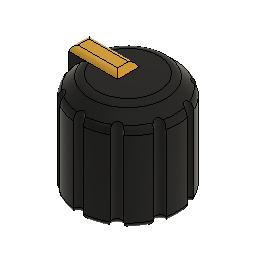
cace_assembly (Autodesk Fusion 360 archive; units mm, degrees)
design "deej knob"
Autodesk Fusion 360 part; units mm, degrees
sketch "Sketch1" plane through (0, 0, 0) normal (0, 0, 1) x (1, 0, 0)
  circle A0 centre (0, 0) radius 3.1
  circle A1 centre (0, 0) radius 5
  circle A2 centre (0, 0) radius 3
  circle A3 centre (0, 5) radius 0.5
  circle A4 centre (-2.9389, 4.0451) radius 0.5
  circle A5 centre (-4.7553, 1.5451) radius 0.5
  circle A6 centre (-4.7553, -1.5451) radius 0.5
  circle A7 centre (-2.9389, -4.0451) radius 0.5
  circle A8 centre (0, -5) radius 0.5
  circle A9 centre (2.9389, -4.0451) radius 0.5
  circle A10 centre (4.7553, -1.5451) radius 0.5
  circle A11 centre (4.7553, 1.5451) radius 0.5
  circle A12 centre (2.9389, 4.0451) radius 0.5
  line L0 (0, 0) -> (0, 1.0451)
  line L1 (0, 1.0451) -> (-4.8896, 1.0451)
  line L2 (0, 0) -> (0, -1.0451)
  line L3 (0, -1.0451) -> (-4.8896, -1.0451)
  dimension "d1" = 6.2
  dimension "d2" = 10
  dimension "d3" = 6
  dimension "d4" = 1
  dimension "d6" = 360
  constraint coincident A0.centre A1.centre
  constraint concentric A0 A1
  constraint concentric A0 A2
  constraint coincident A1 A3.centre
  constraint vertical L0
  constraint horizontal L1
  constraint vertical L2
  constraint horizontal L3
  constraint coincident A1 L1.end
  constraint coincident A1 L3.end
  constraint tangent A6 L3
  constraint tangent A5 L1
  measures "d1" diameter of A0
  measures "d2" diameter of A1
  measures "d3" diameter of A2
  measures "d4" diameter of A3
extrude "Extrude1" add sketch "Sketch1" along normal blind 9 contours A0 A1 A3 A4 A5 A6 A7 A8 A9 A10 A11 A12 L1 L3 | A0 A1 L1 L3 | A1 A5 L1 | A1 A6 L3
extrude "Extrude2" add sketch "Sketch1" along normal blind 9 and the other way blind -4 contours A0 A2 L1 L3 | A0 A2 L1 L3
extrude "Extrude3" add sketch "Sketch1" along normal blind 1 from surface at 9 contours A0 A2 L1 L3 | A0 A1 A3 A4 A5 A6 A7 A8 A9 A10 A11 A12 L1 L3 | A0 A2 L1 L3 | A0 A1 L1 L3 | A2 L0 L1 L2 L3 | A2 L0 L1 L2 L3 | A1 A5 L1 | A1 A6 L3
sketch "Sketch2" plane through (0, 0, 0) normal (1, 0, 0) x (0, 1, 0)
  line L0 (-5.5, 8) -> (-3, 10.5)
  line L1 (-3, 10.5) -> (-5.5, 10.5)
  line L2 (-5.5, 10.5) -> (-5.5, 8)
  dimension "d26" = 8
  dimension "d27" = 3
  constraint horizontal L1
  constraint perpendicular L1 L2
  measures "d26" vertical distance of origin L0.start
  measures "d27" horizontal distance of origin L0.end
revolve "Revolve1" cut sketch "Sketch2" angle 360 about axis through (0, 0, 1.75) along (0, 0, 1)
fillet "Fillet4" radius 1 1 edges at (-1.2657, 3.2631, 10)
fillet "Fillet5" radius 1 10 edges at (4.0451, 2.9389, 8.5) (1.5451, 4.7553, 8.5) (-1.5451, 4.7553, 8.5) (-4.0451, 2.9389, 8.5) (-5, 0, 8.5) (-4.0451, -2.9389, 8.5) (-1.5451, -4.7553, 8.5) (1.5451, -4.7553, 8.5) (4.0451, -2.9389, 8.5) (5, 0, 8.5)
extrude "Extrude4" add sketch "Sketch1" along normal blind 10.5 and the other way blind -7.5 contours A0 A2 L1 L3 | A0 A1 L1 L3 | A2 L0 L1 L2 L3 picked at (-2.8875, 0.9086) picked at (-0.9374, 0.6967)
fillet "Fillet6" radius 0.5 4 edges at (-5, 0, 10.5) (-2.4448, -1.0451, 10.5) (0, 0, 10.5) (-2.4448, 1.0451, 10.5)
fillet "Fillet7" radius 0.5 1 faces at (4.2069, -0.4845, 0)

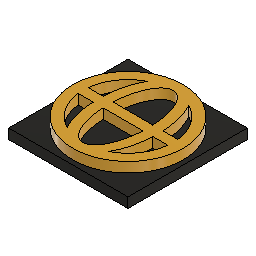
design "www"
Autodesk Fusion 360 part; units mm, degrees
sketch "Sketch1" plane through (0, 0, 0) normal (0, 0, 1) x (1, 0, 0)
  line L0 (5.95, -5.95) -> (-5.95, -5.95)
  line L1 (-5.95, -5.95) -> (-5.95, 5.95)
  line L2 (-5.95, 5.95) -> (5.95, 5.95)
  line L3 (5.95, 5.95) -> (5.95, -5.95)
  line L4 (5.95, -5.95) -> (-5.95, 5.95) construction
  line L5 (-5.95, -5.95) -> (5.95, 5.95) construction
  circle A0 centre (0, 0) radius 5.5
  arc A1 (-2.058, 4.0018) -> (-4.4755, 0.4687) centre (0, 0) ccw
  arc A2 (-4.4755, -0.4687) -> (-2.058, -4.0018) centre (0, 0) ccw
  ellipse E0 centre (0, 0) end of major axis (3, 0) minor radius 5.5 (-2.058, 4.0018) -> (-2.9876, 0.5) ccw
  ellipse E1 centre (0, 0) end of major axis (3, 0) minor radius 5.5 (-2.9876, -0.5) -> (-2.058, -4.0018) ccw
  arc A3 (2.058, -4.0018) -> (4.4721, -0.5) centre (0, 0) ccw
  arc A4 (4.4721, 0.5) -> (2.058, 4.0018) centre (0, 0) ccw
  line L6 (2.9876, 0.5) -> (4.4721, 0.5)
  ellipse E2 centre (0, 0) end of major axis (3, 0) minor radius 5.5 (2.058, -4.0018) -> (2.9876, -0.5) ccw
  ellipse E3 centre (0, 0) end of major axis (3, 0) minor radius 5.5 (2.9876, 0.5) -> (2.058, 4.0018) ccw
  ellipse E4 centre (0, 0) end of major axis (2, 0) minor radius 4.5 (-1.9876, -0.5) -> (1.9876, -0.5) ccw
  ellipse E5 centre (0, 0) end of major axis (2, 0) minor radius 4.5 (1.9876, 0.5) -> (-1.9876, 0.5) ccw
  line L7 (4.4721, -0.5) -> (2.9876, -0.5)
  line L8 (1.9876, -0.5) -> (-1.9876, -0.5)
  line L9 (-2.9876, -0.5) -> (-4.4721, -0.5)
  line L10 (-4.4721, 0.5) -> (-2.9876, 0.5)
  line L11 (-1.9876, 0.5) -> (1.9876, 0.5)
  dimension "d1" = 11.9
  dimension "d2" = 11.9
  constraint horizontal L0
  constraint perpendicular L0 L1
  constraint parallel L0 L2
  constraint parallel L1 L3
  constraint concentric A0 A1
  constraint concentric A0 E0
  constraint concentric A1 A3
  constraint coincident A3.start E0
  constraint concentric E0 E2
  constraint horizontal L7
  constraint parallel L7 L10
  constraint coincident A0.centre A1.centre
  constraint coincident L10.start A1
  constraint coincident L9.end A1
  constraint coincident A2.start A1
  constraint concentric A1 A2
  constraint concentric E0 E1
  constraint coincident L11.start L10
  constraint coincident L8.end L7
  constraint coincident L9.start L7
  constraint coincident A4.start A3
  constraint concentric A3 A4
  constraint coincident L11.end E4
  constraint coincident L6.start E2
  constraint collinear L6 L10
  constraint concentric E2 E3
  constraint coincident L8.start L7
  constraint concentric E4 E5
  constraint collinear L7 L8
  constraint collinear L8 L9
  constraint collinear L10 L11
  measures "d1" distance of L1.end L2.end
  measures "d2" distance of L0.end L1.end
extrude "Extrude1" add sketch "Sketch1" against normal blind 1 contours L0 L1 L2 L3 | A0 | A1 E0 L10 | A2 E1 L9 | A3 E2 L7 | A4 L6 E3 | E4 L8 | E5 L11
extrude "Extrude3" add sketch "Sketch1" along normal blind 1 contours A0

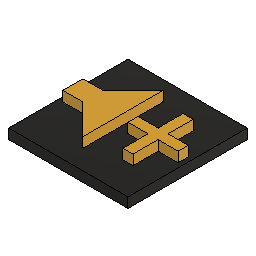
design "volume"
Autodesk Fusion 360 part; units mm, degrees
sketch "Sketch1" plane through (0, 0, 0) normal (0, 0, 1) x (1, 0, 0)
  line L0 (5.95, -5.95) -> (-5.95, -5.95)
  line L1 (-5.95, -5.95) -> (-5.95, 5.95)
  line L2 (-5.95, 5.95) -> (5.95, 5.95)
  line L3 (5.95, 5.95) -> (5.95, -5.95)
  line L4 (5.95, -5.95) -> (-5.95, 5.95) construction
  line L5 (-5.95, -5.95) -> (5.95, 5.95) construction
  line L6 (-0.5, 3.5) -> (-0.5, 0)
  line L7 (0.5, 0) -> (0.5, 0.5)
  line L8 (2.5, 3) -> (3.5, 3)
  line L9 (5.5, 0.5) -> (5.5, -0.5)
  line L10 (3.5, -3) -> (2.5, -3)
  line L11 (0.5, 0) -> (0.5, -0.5)
  line L12 (0.5, 0.5) -> (2.5, 0.5)
  line L13 (2.5, 0.5) -> (2.5, 3)
  line L14 (3.5, 3) -> (3.5, 0.5)
  line L15 (3.5, 0.5) -> (5.5, 0.5)
  line L16 (5.5, -0.5) -> (3.5, -0.5)
  line L17 (3.5, -0.5) -> (3.5, -3)
  line L18 (2.5, -3) -> (2.5, -0.5)
  line L19 (2.5, -0.5) -> (0.5, -0.5)
  line L20 (-0.5, 0) -> (-0.5, -3.5)
  line L21 (-3.5, -1) -> (-5.5, -1)
  line L22 (-5.5, -1) -> (-5.5, 1)
  line L23 (-5.5, 1) -> (-3.5, 1)
  line L24 (-0.5, 3.5) -> (-0.5, 4)
  line L25 (-0.5, 4) -> (-3.5, 1)
  line L26 (-0.5, -3.5) -> (-0.5, -4)
  line L27 (-0.5, -4) -> (-3.5, -1)
  dimension "d1" = 11.9
  dimension "d2" = 11.9
  constraint horizontal L0
  constraint perpendicular L0 L1
  constraint parallel L0 L2
  constraint parallel L1 L3
  constraint coincident L4 origin
  constraint coincident L5 origin
  constraint parallel L1 L7
  constraint perpendicular L7 L12
  constraint perpendicular L8 L13
  constraint perpendicular L9 L15
  constraint perpendicular L9 L16
  constraint perpendicular L10 L17
  constraint perpendicular L10 L18
  constraint perpendicular L11 L19
  constraint parallel L6 L20
  constraint perpendicular L20 L21
  constraint perpendicular L21 L22
  constraint perpendicular L22 L23
  constraint parallel L6 L24
  constraint perpendicular L4 L25
  constraint parallel L24 L26
  constraint perpendicular L5 L27
  measures "d1" distance of L1.end L2.end
  measures "d2" distance of L0.end L1.end
extrude "Extrude1" add sketch "Sketch1" against normal blind 1 contours L0 L1 L2 L3 | L6 L20 L21 L22 L23 L24 L25 L26 L27 | L7 L8 L9 L10 L11 L12 L13 L14 L15 L16 L17 L18 L19
extrude "Extrude2" add sketch "Sketch1" along normal blind 1 contours L6 L20 L21 L22 L23 L24 L25 L26 L27 | L7 L8 L9 L10 L11 L12 L13 L14 L15 L16 L17 L18 L19

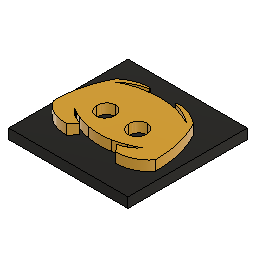
design "discord"
Autodesk Fusion 360 part; units mm, degrees
sketch "Sketch1" plane through (0, 0, 0) normal (0, 0, 1) x (1, 0, 0)
  line L0 (5.95, -5.95) -> (-5.95, -5.95)
  line L1 (-5.95, -5.95) -> (-5.95, 5.95)
  line L2 (-5.95, 5.95) -> (5.95, 5.95)
  line L3 (5.95, 5.95) -> (5.95, -5.95)
  line L4 (5.95, -5.95) -> (-5.95, 5.95) construction
  line L5 (-5.95, -5.95) -> (5.95, 5.95) construction
  spline S0 degree 3 poles (1.569, 0.3676) (1.0713, 0.3676) (0.6784, -0.0602) (0.6784, -0.5928) knots 0 0 0 0 1 1 1 1
  spline S1 degree 3 poles (0.6784, -0.5928) (0.6784, -1.1254) (1.08, -1.5532) (1.569, -1.5532) knots 0 0 0 0 1 1 1 1
  spline S2 degree 3 poles (1.569, -1.5532) (2.0667, -1.5532) (2.4596, -1.1254) (2.4596, -0.5928) knots 0 0 0 0 1 1 1 1
  spline S3 degree 3 poles (2.4596, -0.5928) (2.4596, -0.0602) (2.0579, 0.3676) (1.569, 0.3676) knots 0 0 0 0 1 1 1 1
  spline S4 degree 3 poles (-1.6179, 0.3676) (-2.1156, 0.3676) (-2.5085, -0.0602) (-2.5085, -0.5928) knots 0 0 0 0 1 1 1 1
  spline S5 degree 3 poles (-2.5085, -0.5928) (-2.5085, -1.1254) (-2.1069, -1.5532) (-1.6179, -1.5532) knots 0 0 0 0 1 1 1 1
  spline S6 degree 3 poles (-1.6179, -1.5532) (-1.1202, -1.5532) (-0.7273, -1.1254) (-0.7273, -0.5928) knots 0 0 0 0 1 1 1 1
  spline S7 degree 3 poles (-0.7273, -0.5928) (-0.7186, -0.0602) (-1.1202, 0.3676) (-1.6179, 0.3676) knots 0 0 0 0 1 1 1 1
  spline S8 degree 2 poles (2.4421, -3.6749) (2.1278, -3.2995) (1.8659, -2.9764) knots 0 0 0 1 1 1
  spline S9 degree 2 poles (1.8659, -2.9764) (3.0096, -2.6534) (3.4462, -1.9461) knots 0 0 0 1 1 1
  spline S10 degree 3 poles (3.4462, -1.9461) (3.0882, -2.1819) (2.7477, -2.3478) (2.4421, -2.4613) knots 0 0 0 0 1 1 1 1
  spline S11 degree 3 poles (2.4421, -2.4613) (2.0056, -2.6446) (1.5865, -2.7581) (1.1761, -2.8367) knots 0 0 0 0 1 1 1 1
  spline S12 degree 3 poles (1.1761, -2.8367) (0.3379, -2.9939) (-0.4305, -2.9502) (-1.0853, -2.828) knots 0 0 0 0 1 1 1 1
  spline S13 degree 3 poles (-1.0853, -2.828) (-1.583, -2.7319) (-2.0108, -2.601) (-2.3688, -2.4525) knots 0 0 0 0 1 1 1 1
  spline S14 degree 3 poles (-2.3688, -2.4525) (-2.5696, -2.374) (-2.7879, -2.2779) (-3.0062, -2.1557) knots 0 0 0 0 1 1 1 1
  spline S15 degree 3 poles (-3.0062, -2.1557) (-3.0324, -2.1382) (-3.0586, -2.1295) (-3.0848, -2.112) knots 0 0 0 0 1 1 1 1
  spline S16 degree 3 poles (-3.0848, -2.112) (-3.1022, -2.1033) (-3.111, -2.0946) (-3.1197, -2.0946) knots 0 0 0 0 1 1 1 1
  spline S17 degree 2 poles (-3.1197, -2.0946) (-3.2769, -2.0073) (-3.3642, -1.9461) knots 0 0 0 1 1 1
  spline S18 degree 2 poles (-3.3642, -1.9461) (-2.9451, -2.6359) (-1.8362, -2.9677) knots 0 0 0 1 1 1
  spline S19 degree 2 poles (-1.8362, -2.9677) (-2.0981, -3.2995) (-2.4212, -3.6837) knots 0 0 0 1 1 1
  spline S20 degree 2 poles (-2.4212, -3.6837) (-4.3508, -3.6225) (-5.0842, -2.3652) knots 0 0 0 1 1 1
  spline S21 degree 2 poles (-5.0842, -2.3652) (-5.0842, 0.42) (-3.8269, 2.6814) knots 0 0 0 1 1 1
  spline S22 degree 2 poles (-3.8269, 2.6814) (-2.5696, 3.6157) (-1.3822, 3.5895) knots 0 0 0 1 1 1
  line L6 (-1.3822, 3.5895) -> (-1.2949, 3.4847)
  spline S23 degree 2 poles (-1.2949, 3.4847) (-2.8665, 3.0394) (-3.5824, 2.3496) knots 0 0 0 1 1 1
  spline S24 degree 2 poles (-3.5824, 2.3496) (-3.3904, 2.4544) (-3.0673, 2.5941) knots 0 0 0 1 1 1
  spline S25 degree 3 poles (-3.0673, 2.5941) (-2.1331, 3.0045) (-1.3909, 3.1093) (-1.0853, 3.1442) knots 0 0 0 0 1 1 1 1
  spline S26 degree 3 poles (-1.0853, 3.1442) (-1.0329, 3.1529) (-0.9893, 3.1616) (-0.9369, 3.1616) knots 0 0 0 0 1 1 1 1
  spline S27 degree 3 poles (-0.9369, 3.1616) (-0.4043, 3.2315) (0.1982, 3.249) (0.8268, 3.1791) knots 0 0 0 0 1 1 1 1
  spline S28 degree 3 poles (0.8268, 3.1791) (1.6563, 3.0831) (2.5469, 2.8386) (3.4549, 2.3496) knots 0 0 0 0 1 1 1 1
  spline S29 degree 2 poles (3.4549, 2.3496) (2.7652, 3.0045) (1.2809, 3.4498) knots 0 0 0 1 1 1
  line L7 (1.2809, 3.4498) -> (1.4031, 3.5895)
  spline S30 degree 2 poles (1.4031, 3.5895) (2.5993, 3.6157) (3.8478, 2.6814) knots 0 0 0 1 1 1
  spline S31 degree 2 poles (3.8478, 2.6814) (5.1051, 0.42) (5.1051, -2.3652) knots 0 0 0 1 1 1
  spline S32 degree 3 poles (5.1051, -2.3652) (5.1051, -2.3565) (4.3717, -3.6138) (2.4421, -3.6749) knots 0 0 0 0 1 1 1 1
  dimension "d1" = 11.9
  dimension "d2" = 11.9
  constraint perpendicular L0 L1
  constraint parallel L1 L3
  constraint coincident L4 origin
  constraint coincident L5 origin
  measures "d1" distance of L1.end L2.end
  measures "d2" distance of L0.end L1.end
extrude "Extrude1" add sketch "Sketch1" against normal blind 1 contours L0 L1 L2 L3 | S0 S1 S2 S3 | S4 S5 S6 S7 | S8 S9 S10 S11 S12 S13 S14 S15 S16 S17 S18 S19 S20 S21 S22 L6 S23 S24 S25 S26 S27 S28 S29 L7 S30 S31 S32
extrude "Extrude3" add sketch "Sketch1" along normal blind 1 contours S8 S9 S10 S11 S12 S13 S14 S15 S16 S17 S18 S19 S20 S21 S22 L6 S23 S24 S25 S26 S27 S28 S29 L7 S30 S31 S32

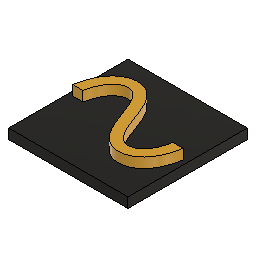
design "system"
Autodesk Fusion 360 part; units mm, degrees
sketch "Sketch1" plane through (0, 0, 0) normal (0, 0, 1) x (1, 0, 0)
  line L0 (5.95, -5.95) -> (-5.95, -5.95)
  line L1 (-5.95, -5.95) -> (-5.95, 5.95)
  line L2 (-5.95, 5.95) -> (5.95, 5.95)
  line L3 (5.95, 5.95) -> (5.95, -5.95)
  line L4 (5.95, -5.95) -> (-5.95, 5.95) construction
  line L5 (-5.95, -5.95) -> (5.95, 5.95) construction
  spline S0 degree 5 poles (-5, 0) (-4.9575, 0.2297) (-4.8598, 0.6679) (-4.6747, 1.2621) (-4.3511, 1.9274) (-3.8228, 2.5423) (-3.1921, 2.9282) (-2.4956, 3.0695) (-1.817, 2.932) (-1.2301, 2.5035) (-0.7463, 1.8241) (-0.3498, 0.9601) (-0.0005, -0.0002) (0.351, -0.9598) (0.7529, -1.8223) (1.2432, -2.5008) (1.8348, -2.9297) (2.5144, -3.0694) (3.2094, -2.9308) (3.8371, -2.5468) (4.3614, -1.9323) (4.6812, -1.266) (4.8631, -0.6702) (4.9587, -0.2305) (5, 0) knots 0 0 0 0 0 0 0.05 0.1 0.15 0.2 0.25 0.3 0.35 0.4 0.45 0.5 0.55 0.6 0.65 0.7 0.75 0.8 0.85 0.9 0.95 1 1 1 1 1 1
  line L6 (-3.5, 3) -> (-1.5, 3)
  line L7 (1.5241, -3) -> (3.5241, -3)
  line L8 (-4.4909, 0) -> (-5.55, 0)
  line L9 (4.4915, 0) -> (5.508, 0)
  spline S1 degree 3 poles (-4.4909, 0) (-4.202, 1.4563) (-3.5685, 2.2271) (-2.8864, 2.4394) (-2.3165, 2.6168) (-1.8076, 2.4436) (-1.3375, 1.7472) (-0.8557, 1.0334) (-0.503, -0.2172) (-0.0186, -1.3122) (0.3354, -2.1125) (0.7938, -2.8423) (1.4733, -3.2241) (2.1901, -3.6268) (3.0825, -3.561) (3.7767, -3.1336) (4.612, -2.6193) (5.1673, -1.6393) (5.4409, -0.3504) (5.4591, -0.2645) (5.4762, -0.1772) (5.4921, -0.0883) (5.4974, -0.0588) (5.5027, -0.0294) (5.508, 0) knots 0.004254 0.004254 0.004254 0.004254 0.210613 0.210613 0.210613 0.38303 0.38303 0.38303 0.559752 0.559752 0.559752 0.688923 0.688923 0.688923 0.82516 0.82516 0.82516 0.989082 0.989082 0.989082 1 1 1 1.008967 1.008967 1.008967 1.008967
  spline S2 degree 3 poles (-5.5085, 0) (-5.5029, 0.0303) (-5.4973, 0.0606) (-5.4917, 0.0909) (-5.2527, 1.3828) (-4.7611, 2.3804) (-3.9943, 2.9693) (-3.3458, 3.4673) (-2.49, 3.6492) (-1.7382, 3.359) (-1.0443, 3.0912) (-0.5365, 2.4519) (-0.1666, 1.7152) (0.3056, 0.7749) (0.6186, -0.3569) (1.0231, -1.1811) (1.3551, -1.8577) (1.7348, -2.2795) (2.1216, -2.4267) (2.7975, -2.684) (3.6536, -2.3065) (4.1588, -1.1313) (4.2954, -0.8137) (4.4079, -0.4363) (4.4915, 0) knots 0 0 0 0 0.009248 0.009248 0.009248 0.168421 0.168421 0.168421 0.30303 0.30303 0.30303 0.427287 0.427287 0.427287 0.585905 0.585905 0.585905 0.716109 0.716109 0.716109 0.943637 0.943637 0.943637 1.005138 1.005138 1.005138 1.005138
  point P0 (-2.5, 3)
  point P1 (2.5241, -3)
  point P2 (5.4921, -0.0883)
  dimension "d1" = 11.9
  dimension "d2" = 11.9
  constraint horizontal L0
  constraint perpendicular L0 L1
  constraint parallel L0 L2
  constraint parallel L1 L3
  constraint coincident L4 origin
  constraint coincident L5 origin
  constraint midpoint P0 L6
  constraint midpoint P1 L7
  constraint horizontal L8
  constraint coincident L8 S2.start
  constraint horizontal L9
  measures "d1" distance of L1.end L2.end
  measures "d2" distance of L0.end L1.end
extrude "Extrude1" add sketch "Sketch1" against normal blind 1 contours L0 L1 L2 L3 | S0 L8 L9 S2 | S0 L8 L9 S1
extrude "Extrude3" add sketch "Sketch1" along normal blind 1 contours S0 L8 L9 S2 | S0 L8 L9 S1

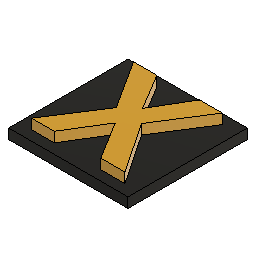
design "active"
Autodesk Fusion 360 part; units mm, degrees
sketch "Sketch1" plane through (0, 0, 0) normal (0, 0, 1) x (1, 0, 0)
  line L0 (5.95, -5.95) -> (-5.95, -5.95)
  line L1 (-5.95, -5.95) -> (-5.95, 5.95)
  line L2 (-5.95, 5.95) -> (5.95, 5.95)
  line L3 (5.95, 5.95) -> (5.95, -5.95)
  line L4 (5.95, -5.95) -> (-5.95, 5.95) construction
  line L5 (-5.95, -5.95) -> (5.95, 5.95) construction
  line L6 (4.6526, -4.9591) -> (2.2411, -4.9591)
  line L7 (2.2411, -4.9591) -> (-0.0749, -1.1921)
  line L8 (-0.0749, -1.1921) -> (-2.391, -4.9591)
  line L9 (-2.391, -4.9591) -> (-4.6526, -4.9591)
  line L10 (-4.6526, -4.9591) -> (-1.3488, 0.1771)
  line L11 (-1.3488, 0.1771) -> (-4.4414, 5)
  line L12 (-4.4414, 5) -> (-2.1117, 5)
  line L13 (-2.1117, 5) -> (0.0341, 1.4169)
  line L14 (0.0341, 1.4169) -> (2.139, 5)
  line L15 (2.139, 5) -> (4.4142, 5)
  line L16 (4.4142, 5) -> (1.2875, 0.0613)
  line L17 (1.2875, 0.0613) -> (4.6526, -4.9591)
  dimension "d1" = 11.9
  dimension "d2" = 11.9
  constraint perpendicular L0 L1
  measures "d1" distance of L1.end L2.end
  measures "d2" distance of L0.end L1.end
extrude "Extrude1" add sketch "Sketch1" against normal blind 1 contours L0 L1 L2 L3 | L6 L7 L8 L9 L10 L11 L12 L13 L14 L15 L16 L17
extrude "Extrude3" add sketch "Sketch1" along normal blind 1 contours L6 L7 L8 L9 L10 L11 L12 L13 L14 L15 L16 L17
